Unifi Switch PSU Mount (Autodesk Fusion 360 design; units mm, degrees)
Autodesk Fusion 360 part; units mm, degrees
sketch "Sketch1" plane through (0, 0, 0) normal (0, 0, 1) x (1, 0, 0)
  line L0 (0, 0) -> (48.5, 0)
  line L1 (48.5, 0) -> (48.5, 20)
  line L2 (48.5, 20) -> (0, 20)
  line L3 (0, 20) -> (0, 0)
  line L4 (0, 0) -> (-3, 0)
  line L5 (-3, 0) -> (-3, 20)
  line L6 (-3, 20) -> (0, 20)
  line L7 (0, 20) -> (0, 0)
  line L8 (48.5, 0) -> (51.5, 0)
  line L9 (51.5, 0) -> (51.5, 20)
  line L10 (51.5, 20) -> (48.5, 20)
  line L11 (48.5, 20) -> (48.5, 0)
  line L12 (-3, 0) -> (-18, 0)
  line L13 (-18, 0) -> (-18, 20)
  line L14 (-18, 20) -> (-3, 20)
  line L15 (-3, 20) -> (-3, 0)
  line L16 (51.5, 0) -> (66.5, 0)
  line L17 (66.5, 0) -> (66.5, 20)
  line L18 (66.5, 20) -> (51.5, 20)
  line L19 (51.5, 20) -> (51.5, 0)
  line L20 (51.5, 0) -> (66.5, 0)
  line L21 (66.5, 0) -> (66.5, 2.5)
  line L22 (66.5, 2.5) -> (51.5, 2.5)
  line L23 (51.5, 2.5) -> (51.5, 0)
  line L24 (51.5, 20) -> (66.5, 20)
  line L25 (66.5, 20) -> (66.5, 17.5)
  line L26 (66.5, 17.5) -> (51.5, 17.5)
  line L27 (51.5, 17.5) -> (51.5, 20)
  line L28 (-3, 0) -> (-18, 0)
  line L29 (-18, 0) -> (-18, 2.5)
  line L30 (-18, 2.5) -> (-3, 2.5)
  line L31 (-3, 2.5) -> (-3, 0)
  line L32 (-3, 20) -> (-18, 20)
  line L33 (-18, 20) -> (-18, 17.5)
  line L34 (-18, 17.5) -> (-3, 17.5)
  line L35 (-3, 17.5) -> (-3, 20)
  circle A0 centre (59, 10) radius 2
  circle A1 centre (-10.5, 10) radius 2
  line L36 (11.75, 0) -> (36.75, 0)
  line L37 (36.75, 0) -> (36.75, -3)
  line L38 (36.75, -3) -> (11.75, -3)
  line L39 (11.75, -3) -> (11.75, 0)
  dimension "d1" = 48.5
  dimension "d2" = 20
  dimension "d3" = 3
  dimension "d4" = 3
  dimension "d5" = 15
  dimension "d6" = 15
  dimension "d7" = 2.5
  dimension "d8" = 2.5
  dimension "d9" = 2.5
  dimension "d10" = 2.5
  dimension "d11" = 4
  dimension "d12" = 4
  dimension "d13" = 25
  dimension "d14" = 3
  dimension "d15" = 11.75
  constraint horizontal L0
  constraint vertical L1
  constraint horizontal L2
  constraint vertical L3
  constraint coincident L0.start L3.end
  constraint horizontal L4
  constraint vertical L5
  constraint horizontal L6
  constraint vertical L7
  constraint horizontal L8
  constraint vertical L9
  constraint horizontal L10
  constraint vertical L11
  constraint horizontal L12
  constraint vertical L13
  constraint horizontal L14
  constraint vertical L15
  constraint horizontal L16
  constraint vertical L17
  constraint horizontal L18
  constraint vertical L19
  constraint horizontal L20
  constraint vertical L21
  constraint horizontal L22
  constraint vertical L23
  constraint horizontal L24
  constraint vertical L25
  constraint horizontal L26
  constraint vertical L27
  constraint horizontal L28
  constraint vertical L29
  constraint horizontal L30
  constraint vertical L31
  constraint horizontal L32
  constraint vertical L33
  constraint horizontal L34
  constraint vertical L35
  constraint horizontal L36
  constraint vertical L37
  constraint horizontal L38
  constraint vertical L39
  constraint coincident L0 L36.start
  measures "d1" distance of L0.start L0.end
  measures "d2" distance of L0.start L2.end
  measures "d3" distance of L0.start L4.end
  measures "d4" distance of L0.end L8.end
  measures "d5" distance of L4.end L12.end
  measures "d6" distance of L8.end L16.end
  measures "d7" distance of L8.end L22.end
  measures "d8" distance of L9.end L26.end
  measures "d9" distance of L4.end L30.end
  measures "d10" distance of L5.end L34.end L0.end
  measures "d11" diameter of A0
  measures "d12" diameter of A1
  measures "d13" distance of L36.start L36.end
  measures "d14" distance of L36.start L38.end
  measures "d15" distance of L11 L36.end
extrude "Extrude1" add sketch "Sketch1" along normal blind 2.5 contours L5 L12 L13 L15 L28 L29 L30 L31 | L5 L13 L14 L15 L32 L33 L34 L35 | L5 L13 L15 L30 L34 | L9 L17 L18 L19 L24 L25 L26 L27 | L9 L16 L17 L19 L20 L21 L22 L23 | L9 L17 L19 L22 L26 makes body 1 at (-10.4502, 2.6685, 0) makes body 2 at (59.0498, 2.6685, 0)
extrude "Extrude2" add sketch "Sketch1" along normal blind 35 contours L3 L4 L5 L6 L7 L15 L31 L35 | L1 L8 L9 L10 L11 L19 L23 L27 bodies 1 2
extrude "Extrude3" add sketch "Sketch1" along normal blind 2.5 from surface at 32.5 contours L0 L1 L2 L3 L7 L11 L36 bodies 1 2
extrude "Extrude4" add sketch "Sketch1" along normal blind 18 contours L5 L12 L13 L15 L28 L29 L30 L31 | L5 L13 L14 L15 L32 L33 L34 L35 | L9 L17 L18 L19 L24 L25 L26 L27 | L9 L16 L17 L19 L20 L21 L22 L23 bodies 1
chamfer "Chamfer1" distance 15 angle 45 4 edges at (-18, 18.75, 18) (-18, 1.25, 18) (66.5, 18.75, 18) (66.5, 1.25, 18) on bodies 1
fillet "Fillet1" radius 2 2 edges at (-3, 10, 35) (51.5, 10, 35) on bodies 1
copy_body "CopyPasteBodies1" bodies 1 makes body 3
move_body "Move1" bodies 3 to x (1, 0, 0) y (0, 1, 0) z (0, 0, 1) at (0, 70, 0)
extrude "Extrude5" add sketch "Sketch1" along normal blind 10 from surface at 25 contours L0 L36 L37 L38 L39 bodies 1
